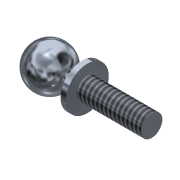
# Autodesk Inventor part: Tripod_BallShaft
Saved by Autodesk Inventor 2014 (Build 180170000, 170)
## iProperties
Created: 2012-06-04
Part Number: Tripod_BallShaft
Material: Polypropylene
Document SubType Name: Modeling
Designer: Lee
Density: 0.899 g/cm^3
Mass: 1.71929 g
Surface Area: 12.1444 cm^2
Volume: 1.91245 cm^3
Appearance: Plastic-Silver
Author: Lee
Autodesk Inventor part; units mm, degrees
ref_plane "YZ Plane" through (0, 0, 0) normal (1, 0, 0) x (0, 1, 0)
ref_plane "XZ Plane" through (0, 0, 0) normal (0, 1, 0) x (-1, 0, 0)
ref_plane "XY Plane" through (0, 0, 0) normal (0, 0, 1) x (1, 0, 0)
sketch "Sketch1" plane through (0, 0, 0) normal (0, 0, 1) x (1, 0, 0)
  line L0 (-9.4288, 0) -> (41.915, 0)
  line L1 (30.1625, 0) -> (30.1625, 3.175)
  line L2 (30.1625, 3.175) -> (11.1125, 3.175)
  line L3 (11.1125, 3.175) -> (11.1125, 6.35)
  line L4 (11.1125, 6.35) -> (9.525, 6.35)
  line L5 (9.525, 6.35) -> (9.525, 2.962)
  line L6 (8.255, 1.692) -> (7.0207, 1.692)
  arc A0 (5.8506, 2.4684) -> (-6.35, 0) centre (0, 0) ccw
  arc A1 (5.8506, 2.4684) -> (7.0207, 1.692) centre (7.0207, 2.962) ccw
  arc A2 (8.255, 1.692) -> (9.525, 2.962) centre (8.255, 2.962) ccw
  line L7 (-6.35, 0) -> (30.1625, 0)
  dimension "d0" = 1.27
  dimension "d1" = 9.525
  dimension "d3" = 12.7
  dimension "d4" = 6.35
  dimension "d5" = 12.7
  dimension "d6" = 1.5875
  dimension "d7" = 19.05
  constraints: 16 end point, 6 point on circle, 5 parallel, 4 tangent, 3 centre point, 2 perpendicular, 1 coincident, 1 equal radius, 1 point on line
  measures "d0" radius of A1
  measures "d1" distance from line of L5 point (0, 0)
  measures "d4" diameter of L2 L0
  measures "d5" diameter of L4 L0
  measures "d6" distance of L3.end L4.end
  measures "d7" distance between parallel lines of L1 L3
revolve "Revolution1" add sketch "Sketch1" angle 360 about axis through (-9.4288, 0, 0) along (1, 0, 0)
thread "Thread1" size "1/4-20 UNC" class "2A" standard "ANSI Unified Screw Threads" full length
body "Solid1"
